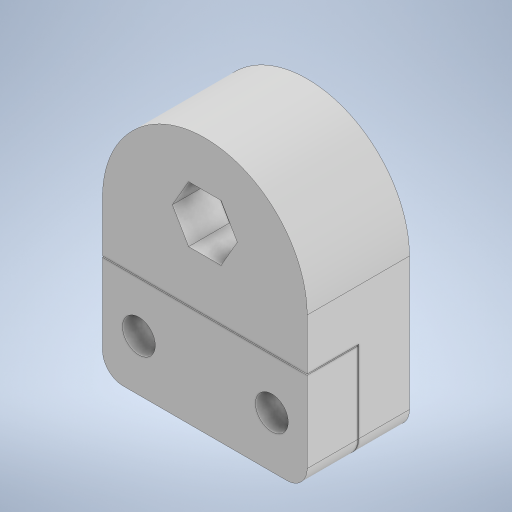
# Autodesk Inventor part: Y Outrigger
Saved by Autodesk Inventor 2023.1 (Build 271208000, 208)
## iProperties
Created: 2022-11-07
Part Number: Y Outrigger
Material: Generic
Document SubType Name: Modeling
Designer: nicol
Density: 1 g/cm^3
Appearance: Default
Author: nicol
Autodesk Inventor part; units mm, degrees
ref_plane "YZ Plane" through (0, 0, 0) normal (1, 0, 0) x (0, 1, 0)
ref_plane "XZ Plane" through (0, 0, 0) normal (0, 1, 0) x (-1, 0, 0)
ref_plane "XY Plane" through (0, 0, 0) normal (0, 0, 1) x (1, 0, 0)
sketch "Sketch1" plane through (0, 0, 0) normal (0, 0, 1) x (1, 0, 0)
  line L0 (0, 0) -> (20, 0)
  line L1 (20, 0) -> (20, 15)
  line L2 (20, 15) -> (0, 15)
  line L3 (0, 15) -> (0, 0)
  arc A0 (20, 15) -> (0, 15) centre (10, 15) ccw
  dimension "d0" = 20
  dimension "d1" = 15
  constraints: 8 end point, 2 parallel, 2 point on circle, 1 centre point, 1 horizontal, 1 midpoint, 1 perpendicular
  measures "d0" distance of L0.start L0.end
  measures "d1" distance of L0.end L1.end
extrude "Extrusion1" add sketch "Sketch1" along normal blind 10
sketch "Sketch2" plane through (0, 0, 0) normal (0, -1, 0) x (1, 0, 0)
  circle A0 centre (10, 5) radius 2.5
  line L0 (0, 0) -> (20, 0) projected
  line L1 (20, 0) -> (20, 10) projected
  line L2 (0, 10) -> (20, 10) projected
  line L3 (0, 0) -> (0, 10) projected
  point P0 (20, 5)
  point P1 (10, 10)
  dimension "d4" = 5
  constraints: 2 midpoint, 1 centre point, 1 horizontal alignment, 1 vertical alignment
  measures "d4" diameter of A0
extrude "Extrusion2" cut sketch "Sketch2" against normal blind 10 contours A0
sketch "Sketch3" plane through (0, 0, 10) normal (0, 0, 1) x (1, 0, 0)
  line L0 (12.5, 10) -> (7.5, 10) projected
  line L1 (12.5, 0) -> (7.5, 0) projected
  line L2 (12.5, 10) -> (7.5, 10) construction
  line L3 (7.5, 10) -> (12.5, 10) construction
  line L4 (12.5, 10) -> (12.5, 0) construction
  line L5 (12.5, 0) -> (7.5, 0) construction
  line L6 (7.5, 0) -> (7.5, 10) construction
  line L7 (3.55, 1.8246) -> (0.8, 3.4123)
  line L8 (0.8, 3.4123) -> (0.8, 6.5877)
  line L9 (0.8, 6.5877) -> (3.55, 8.1754)
  line L10 (3.55, 8.1754) -> (6.3, 6.5877)
  line L11 (6.3, 6.5877) -> (6.3, 3.4123)
  line L12 (6.3, 3.4123) -> (3.55, 1.8246)
  line L13 (16.55, 1.8246) -> (13.8, 3.4123)
  line L14 (13.8, 3.4123) -> (13.8, 6.5877)
  line L15 (13.8, 6.5877) -> (16.55, 8.1754)
  line L16 (16.55, 8.1754) -> (19.3, 6.5877)
  line L17 (19.3, 6.5877) -> (19.3, 3.4123)
  line L18 (19.3, 3.4123) -> (16.55, 1.8246)
  point P0 (0, 0)
  point P1 (3.55, 5)
  point P2 (16.55, 5)
  point P3 (6.3, 5)
  point P4 (7.5, 5)
  point P5 (13.8, 5)
  point P6 (12.5, 5)
  dimension "d7" = 5.5
  dimension "d8" = 5.5
  dimension "d9" = 1.3
  dimension "d10" = 1.2
  constraints: 32 end point, 4 midpoint, 4 parallel, 2 horizontal alignment, 1 horizontal, 1 perpendicular, 26 other
  measures "d7" distance between parallel lines of L16 L13
  measures "d8" distance between parallel lines of L7 L10
  measures "d9" distance between parallel lines of L4 L14
  measures "d10" distance between parallel lines of L6 L11
hole "Hole1" at (3.55, 5, 10) at (16.55, 5, 10) direction (0, 0, -1) diameter 3.2 end through all
extrude "Extrusion3" cut sketch "Sketch3" along normal blind 3 from surface at -10
sketch "Sketch4" plane through (20, 0, 0) normal (1, 0, 0) x (0, 0, -1)
  line L0 (-2.5, 10) -> (-7.5, 10) projected
  line L1 (-2.5, 0) -> (-7.5, 0) projected
  line L2 (-2.5, 10) -> (-7.5, 10) construction
  line L3 (-7.5, 10) -> (-2.5, 10) construction
  line L4 (-2.5, 10) -> (-2.5, 0) construction
  line L5 (-2.5, 0) -> (-7.5, 0) construction
  line L6 (-7.5, 0) -> (-7.5, 10) construction
  line L7 (-10, 10) -> (-4.95, 10)
  line L8 (-4.95, 10) -> (-4.95, 0)
  line L9 (-4.95, 0) -> (-5.05, 0)
  line L10 (-5.05, 0) -> (-5.05, 9.9)
  line L11 (-5.05, 9.9) -> (-10, 9.9)
  line L12 (-10, 9.9) -> (-10, 10)
  line L13 (-10, 0) -> (-10, 15) projected
  line L14 (0, 0) -> (-10, 0) projected
  point P0 (-5, 0)
  point P1 (-5, 0)
  point P2 (-4.95, 0)
  point P3 (-4.95, 10)
  dimension "d20" = 0.1
  constraints: 20 end point, 4 perpendicular, 3 collinear, 2 horizontal, 2 midpoint, 2 parallel, 2 vertical, 1 coincident
  measures "d20" distance of L8.end L9.end
extrude "Extrusion4" cut sketch "Sketch4" against normal through all contours L8 L1 L10 L11 L12 L7 L0
sketch "Sketch5" plane through (0, 0, 10) normal (0, 0, 1) x (1, 0, 0)
  line L0 (11.5877, 15) -> (8.4123, 15)
  line L1 (8.4123, 15) -> (6.8246, 17.75)
  line L2 (6.8246, 17.75) -> (8.4123, 20.5)
  line L3 (8.4123, 20.5) -> (11.5877, 20.5)
  line L4 (11.5877, 20.5) -> (13.1754, 17.75)
  line L5 (13.1754, 17.75) -> (11.5877, 15)
  arc A0 (20, 15) -> (0, 15) centre (10, 15) ccw projected
  point P0 (0, 0)
  point P1 (10, 17.75)
  dimension "d23" = 5.5
  constraints: 12 end point, 1 horizontal, 1 midpoint, 1 vertical alignment, 13 other
  measures "d23" distance between parallel lines of L0 L3
extrude "Extrusion5" cut sketch "Sketch5" against normal blind 4
hole "Hole2" at (10, 17.75, 10) direction (0, 0, -1) diameter 3.2 end through all
chamfer "Chamfer1" distance 0.5 angle 45 4 edges at (7.5005, 5, 4.95) (7.5005, 4.95, 5.05) (12.4995, 5, 4.95) (12.4995, 4.95, 5.05)
fillet "Fillet1" radius 2 4 edges at (0, 0, 2.475) (20, 0, 2.475) (20, 0, 7.525) (0, 0, 7.525)
sketch "Sketch6" plane through (0, 0, 0) normal (0, 0, -1) x (-1, 0, 0)
  circle A0 centre (-16.55, 5) radius 1.6 projected
  line L0 (-19.3, 3.4123) -> (-16.55, 1.8246) projected
  line L1 (-16.55, 1.8246) -> (-13.8, 3.4123) projected
  line L2 (-13.8, 3.4123) -> (-13.8, 6.5877) projected
  line L3 (-13.8, 6.5877) -> (-16.55, 8.1754) projected
  line L4 (-16.55, 8.1754) -> (-19.3, 6.5877) projected
  line L5 (-19.3, 6.5877) -> (-19.3, 3.4123) projected
  circle A1 centre (-3.55, 5) radius 1.6 projected
  line L6 (-6.3, 3.4123) -> (-3.55, 1.8246) projected
  line L7 (-3.55, 1.8246) -> (-0.8, 3.4123) projected
  line L8 (-0.8, 3.4123) -> (-0.8, 6.5877) projected
  line L9 (-0.8, 6.5877) -> (-3.55, 8.1754) projected
  line L10 (-3.55, 8.1754) -> (-6.3, 6.5877) projected
  line L11 (-6.3, 6.5877) -> (-6.3, 3.4123) projected
  line L12 (-5.15, 6.6) -> (-1.95, 6.6)
  line L13 (-1.95, 7.2517) -> (-1.95, 2.7483)
  line L14 (-1.95, 3.4) -> (-5.15, 3.4)
  line L15 (-5.15, 2.7483) -> (-5.15, 7.2517)
  line L16 (-5.15, 6.6) -> (-1.95, 3.4) construction
  line L17 (-1.95, 6.6) -> (-5.15, 3.4) construction
  line L18 (-18.15, 6.6) -> (-14.95, 6.6)
  line L19 (-14.95, 7.2517) -> (-14.95, 2.7483)
  line L20 (-14.95, 3.4) -> (-18.15, 3.4)
  line L21 (-18.15, 2.7483) -> (-18.15, 7.2517)
  line L22 (-18.15, 6.6) -> (-14.95, 3.4) construction
  line L23 (-14.95, 6.6) -> (-18.15, 3.4) construction
  point P0 (0, 0)
  point P1 (-14.95, 5)
  point P2 (-16.55, 6.6)
  point P3 (-16.55, 3.4)
  point P4 (-18.15, 5)
  point P5 (-5.15, 5)
  point P6 (-3.55, 6.6)
  point P7 (-3.55, 3.4)
  point P8 (-1.95, 5)
  constraints: 24 end point, 17 point on line, 4 midpoint, 4 parallel, 3 tangent, 2 horizontal, 2 perpendicular
extrude "Extrusion6" cut sketch "Sketch6" against normal blind 0.15 from surface at -3 contours A0 | L19 L20 A0 | A0 L18 L19 | A0 L21 L18 | L18 L21 L4 L3 L19 | L20 L21 A0 | L20 L19 L1 L0 L21 | A1 | L13 L14 A1 | A1 L12 L13 | A1 L15 L12 | L12 L15 L10 L9 L13 | L14 L15 A1 | L14 L13 L7 L6 L15
extrude "Extrusion7" cut sketch "Sketch6" against normal blind 0.15 from surface at -3.15 contours L19 L20 A0 | A0 L18 L19 | A0 L21 L18 | L20 L21 A0 | L13 L14 A1 | A1 L12 L13 | A1 L15 L12 | L14 L15 A1
body "Solid1"
